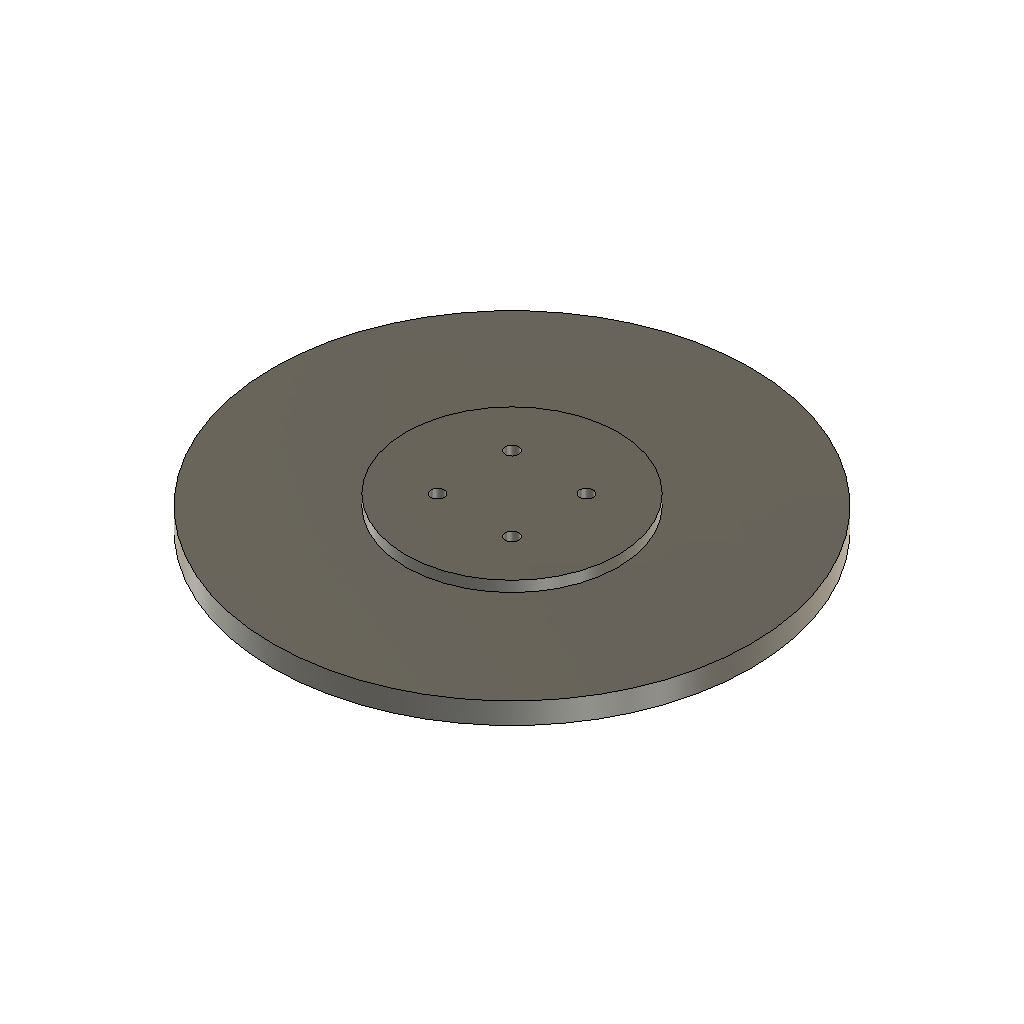
Rotor (Autodesk Fusion 360 design; units mm, degrees)
Autodesk Fusion 360 part; units mm, degrees
sketch "Base" plane through (0, 0, 0) normal (0, 0, 1) x (1, 0, 0)
  circle A0 centre (0, 0) radius 45
  dimension "d1" = 90
  constraint coincident A0.centre origin
  measures "d1" diameter of A0
extrude "Extrude1" add sketch "Base" along normal blind 4
sketch "Stand" plane through (0, 0, 4) normal (0, 0, 1) x (-1, 0, 0)
  circle A0 centre (0, 0) radius 45
  circle A1 centre (0, 0) radius 20
  dimension "d4" = 40
  constraint coincident A0.centre A1.centre
  measures "d4" diameter of A1
extrude "Extrude2" add sketch "Stand" along normal blind 2 contours A1
sketch "Holes" plane through (0, 0, 6) normal (0, 0, 1) x (-1, 0, 0)
  circle A0 centre (0, 0) radius 20
  circle A1 centre (7, -7) radius 1.25
  circle A2 centre (-7, -7) radius 1.25
  line L0 (20, 0) -> (20, -20)
  line L1 (20, -20) -> (0, -20)
  line L2 (-20, 0) -> (-20, 20)
  line L3 (-20, 20) -> (0, 20)
  line L4 (20, -20) -> (-20, -20)
  line L5 (-20, -20) -> (-20, 20)
  line L6 (-20, 20) -> (20, 20)
  line L7 (20, 20) -> (20, -20)
  circle A3 centre (7, 7) radius 1.25
  circle A4 centre (-7, 7) radius 1.25
  dimension "d7" = 2.5
  dimension "d8" = 2.5
  dimension "d10" = 13
  dimension "d11" = 13
  dimension "d12" = 13
  dimension "d13" = 13
  dimension "d14" = 2.5
  dimension "d15" = 2.5
  dimension "d16" = 13
  dimension "d17" = 13
  dimension "d18" = 13
  dimension "d19" = 13
  constraint vertical L0
  constraint horizontal L1
  constraint vertical L2
  constraint horizontal L3
  constraint horizontal L4
  constraint vertical L5
  constraint horizontal L6
  constraint vertical L7
  measures "d7" diameter of A1
  measures "d8" diameter of A2
  measures "d10" distance of A1.centre L7
  measures "d11" distance of A1.centre L1
  measures "d12" distance of A2.centre L4
  measures "d13" distance of A2.centre L5
  measures "d14" diameter of A3
  measures "d15" diameter of A4
  measures "d16" distance of L7 A3.centre
  measures "d17" distance of L2 A4.centre
  measures "d18" distance of L6 A3.centre
  measures "d19" distance of L6 A4.centre
extrude "Extrude3" cut sketch "Holes" against normal blind 6 contours A1 | A2 | A3 | A4
sketch "Fillets" plane through (0, 0, 0) normal (0, 0, -1) x (1, 0, 0)
  circle A0 centre (7, -7) radius 1.25
  circle A1 centre (-7, 7) radius 1.25
  circle A2 centre (-7, -7) radius 1.25
  circle A3 centre (7, 7) radius 1.25
  circle A4 centre (0, 0) radius 45
  circle A5 centre (-7, 7) radius 2
  circle A6 centre (7, 7) radius 2
  circle A7 centre (-7, -7) radius 2
  circle A8 centre (7, -7) radius 2
  dimension "d27" = 4
  dimension "d28" = 4
  dimension "d29" = 4
  dimension "d30" = 4
  constraint concentric A1 A5
  constraint concentric A3 A6
  constraint concentric A2 A7
  constraint concentric A0 A8
  measures "d27" diameter of A5
  measures "d28" diameter of A6
  measures "d29" diameter of A7
  measures "d30" diameter of A8
extrude "Extrude5" cut sketch "Fillets" against normal blind 2 contours A5 | A6 | A7 | A8
